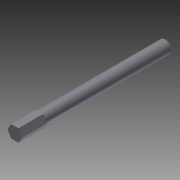
# Autodesk Inventor part: wheel shaft
Saved by Autodesk Inventor 2012 (Build 160160000, 160)
## iProperties
Created: 2012-02-07
Part Number: wheel shaft
Material: Steel
Document SubType Name: Modeling
Designer: Antonella Wilby
Density: 7.85 g/cm^3
Mass: 154.142 g
Surface Area: 64.6389 cm^2
Volume: 19.6359 cm^3
Author: Antonella Wilby
Autodesk Inventor part; units mm, degrees
ref_plane "YZ Plane" through (0, 0, 0) normal (1, 0, 0) x (0, 1, 0)
ref_plane "XZ Plane" through (0, 0, 0) normal (0, 1, 0) x (-1, 0, 0)
ref_plane "XY Plane" through (0, 0, 0) normal (0, 0, 1) x (1, 0, 0)
sketch "Sketch1" plane through (0, 0, 0) normal (0, 0, 1) x (1, 0, 0)
  line L0 (3.6662, 6.35) -> (7.3323, 0)
  line L1 (7.3323, 0) -> (3.6662, -6.35)
  line L2 (3.6662, -6.35) -> (-3.6662, -6.35)
  line L3 (-3.6662, -6.35) -> (-7.3323, 0)
  line L4 (-7.3323, 0) -> (-3.6662, 6.35)
  line L5 (-3.6662, 6.35) -> (3.6662, 6.35)
  point P0 (0, 0)
  point P1 (0, 0)
  point P2 (0, 6.35)
  dimension "d0" = 12.7
  constraints: 12 end point, 1 coincident, 1 midpoint, 1 vertical alignment, 13 other
  measures "d0" distance between parallel lines of L5 L2
extrude "Extrusion1" add sketch "Sketch1" along normal mid plane 152.4
sketch "Sketch2" plane through (0, 0, -76.2) normal (0, 0, -1) x (-1, 0, 0)
  line L0 (-3.6662, 6.35) -> (3.6662, 6.35) projected
  line L1 (-7.3323, 0) -> (-3.6662, 6.35) projected
  line L2 (-3.6662, -6.35) -> (-7.3323, 0) projected
  line L3 (3.6662, -6.35) -> (-3.6662, -6.35) projected
  line L4 (7.3323, 0) -> (3.6662, -6.35) projected
  line L5 (3.6662, 6.35) -> (7.3323, 0) projected
  circle A0 centre (0, 0) radius 6.35
  constraints: 1 centre point, 1 coincident, 1 tangent
extrude "Extrusion2" cut sketch "Sketch2" against normal blind 127 contours L0 A0 L1 | L0 L5 A0 | A0 L2 L1 | L5 L4 A0 | A0 L3 L2 | A0 L4 L3
body "Solid1"
